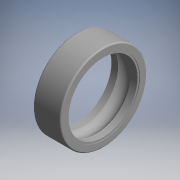
# Autodesk Inventor part: 607ZZ Outer ring
Saved by Autodesk Inventor 2017.3 (Build 213256000, 256)
## iProperties
Part Number: 607ZZ Outer ring
Material: Generic
Catalog Web Link: www.cadenas.de
Description: Six types or-Metric system sizes
Vendor: NTN
Document SubType Name: Modeling
Designer: partserver
Manufacturer: NTN
Mass: 0.543098 g
Surface Area: 8.65362 cm^2
Volume: 0.543098 cm^3
Density: 1 g/cm^3
Appearance: PSOLRGB-192-192-192
Category: PARTsolutions
Company: NTN
Title: 607ZZ Outer ring
Author: Cadenas PARTsolutions
Comments: Metric system sizes
PSOL_IDENT_0: {$CADENAS_DATA\23d-libs\ntn\ball_roller_bearings\miniature_extra_small_bb\metric_system_sizes\mss_or
PSOL_IDENT_1: .prj},181 {VTYP=3D},{NB=607ZZ Outer ring},{LINA=607ZZ Outer ring},{NN=Six types or},{DATE=21.12.2021
PSOL_IDENT_2: 04:23:05},{GEOMDATE=06.03.2020 10:07:12},{VERSION=},{LINEID=12950},{WBVAR=},{WBNUMERIC=}  {NB=607ZZ
PSOL_IDENT_3: Outer ring},{LINA=607ZZ Outer ring},{KT=DUMMY},{IDNR=},{SD=7.0},{D=19},{B=6.0},{R=0.30},{ORDER=607Z
PSOL_IDENT_4: Z},{CR=2 240},{COR=910},{CRF=228},{CORF=93},{LSG=34 000},{LSO=40 000},{MASS=8.00},{D1=0.0},{D2=0.0},
PSOL_IDENT_5: {C1=0.0},{C2=0.0},{ORDER1=607},{WSS=607ZZ},{WDS=ZZ},{UTWF=0},{FORSS=0},{FORDS=0},{DA1=9},{DA2=10,4},
PSOL_IDENT_6: {DA=17},{RAS=0,3},{MASS1=0.00},{B1=6.0},{VERS=3},{X=6},{N=7},{O=40.82},{RB=1.776}
NB: 607ZZ Outer ring
NN: Six types or
NT: Metric system sizes
NBSYN: $ORDER. Outer ring
LINA: 607ZZ Outer ring
CATALOG: NTN Corporation
SD: 7
D: 19
B: 6
R: 0.3
CR: 2 240
COR: 910
CRF: 228
CORF: 93
LSG: 34 000
LSO: 40 000
MASS: 8
D1: 0
D2: 0
C1: 0
C2: 0
ORDER1: 607
WSS: 607ZZ
WDS: ZZ
UTWF: 0
FORSS: 0
FORDS: 0
DA1: 9
DA2: 10,4
DA: 17
RAS: 0,3
MASS1: 0
B1: 6
VERS: 3
SUPPLIER: NTN
ARTICLENO: 607ZZ Outer ring
BOMINFO: 607ZZ Outer ring
CREATOR: CADENAS GmbH
Autodesk Inventor part; units mm, degrees
sketch "Sketch_3" plane through (0, 0, 0) normal (0, 0, 1) x (1, 0, 0)
  line L0 (6, 0) -> (0, 0)
  line L1 (0, 7.964) -> (0.135, 7.964)
  line L2 (0.135, 7.964) -> (0.135, 7.58)
  line L3 (0.135, 7.58) -> (1.5901, 7.58)
  arc A0 (4.4099, 7.58) -> (1.5901, 7.58) centre (3, 6.5) ccw
  line L4 (4.4099, 7.58) -> (5.865, 7.58)
  line L5 (5.865, 7.58) -> (5.865, 7.964)
  line L6 (5.865, 7.964) -> (6, 7.964)
  line L7 (6, 7.964) -> (6, 9.2)
  arc A1 (6, 9.2) -> (5.7, 9.5) centre (5.7, 9.2) ccw
  line L8 (5.7, 9.5) -> (0.3, 9.5)
  arc A2 (0.3, 9.5) -> (0, 9.2) centre (0.3, 9.2) ccw
  line L9 (0, 9.2) -> (0, 7.964)
  constraints: 20 end point, 6 point on circle, 3 centre point
revolve "Revolution1" add sketch "Sketch_3" angle 360 about axis through (6, 0, 0) along (1, 0, 0)
ref_plane "mss_or_XY" through (0, 0, 0) normal (1, 0, 0) x (0, 0, -1)
ref_plane "mss_or_YZ" through (0, 0, 0) normal (0, 0, -1) x (0, 1, 0)
ref_plane "mss_or_ZX" through (0, 0, 0) normal (0, 1, 0) x (1, 0, 0)
ref_plane "mss_or11_XY" through (6, 0, 0) normal (1, 0, 0) x (0, 0, -1)
ref_plane "mss_or11_YZ" through (6, 0, 0) normal (0, 0, -1) x (0, 1, 0)
ref_plane "mss_or11_ZX" through (6, 0, 0) normal (0, 1, 0) x (1, 0, 0)
ref_plane "mss_or2_1_XY" through (3, 6.5, 0) normal (1, 0, 0) x (0, 0, -1)
ref_plane "mss_or2_1_YZ" through (3, 6.5, 0) normal (0, 0, -1) x (0, 1, 0)
ref_plane "mss_or2_1_ZX" through (3, 6.5, 0) normal (0, 1, 0) x (1, 0, 0)
ref_plane "mss_or2_2_XY" through (3, 4.0527, 5.0819) normal (1, 0, 0) x (0, 0, -1)
ref_plane "mss_or2_2_YZ" through (3, 4.0527, 5.0819) normal (0, 0, -1) x (0, 1, 0)
ref_plane "mss_or2_2_ZX" through (3, 4.0527, 5.0819) normal (0, 1, 0) x (1, 0, 0)
ref_plane "mss_or2_3_XY" through (3, -1.4464, 6.337) normal (1, 0, 0) x (0, 0, -1)
ref_plane "mss_or2_3_YZ" through (3, -1.4464, 6.337) normal (0, 0, -1) x (0, 1, 0)
ref_plane "mss_or2_3_ZX" through (3, -1.4464, 6.337) normal (0, 1, 0) x (1, 0, 0)
ref_plane "mss_or2_4_XY" through (3, -5.8563, 2.8202) normal (1, 0, 0) x (0, 0, -1)
ref_plane "mss_or2_4_YZ" through (3, -5.8563, 2.8202) normal (0, 0, -1) x (0, 1, 0)
ref_plane "mss_or2_4_ZX" through (3, -5.8563, 2.8202) normal (0, 1, 0) x (1, 0, 0)
ref_plane "mss_or2_5_XY" through (3, -5.8563, -2.8202) normal (1, 0, 0) x (0, 0, -1)
ref_plane "mss_or2_5_YZ" through (3, -5.8563, -2.8202) normal (0, 0, -1) x (0, 1, 0)
ref_plane "mss_or2_5_ZX" through (3, -5.8563, -2.8202) normal (0, 1, 0) x (1, 0, 0)
ref_plane "mss_or2_6_XY" through (3, -1.4464, -6.337) normal (1, 0, 0) x (0, 0, -1)
ref_plane "mss_or2_6_YZ" through (3, -1.4464, -6.337) normal (0, 0, -1) x (0, 1, 0)
ref_plane "mss_or2_6_ZX" through (3, -1.4464, -6.337) normal (0, 1, 0) x (1, 0, 0)
ref_plane "mss_or2_7_XY" through (3, 4.0527, -5.0819) normal (1, 0, 0) x (0, 0, -1)
ref_plane "mss_or2_7_YZ" through (3, 4.0527, -5.0819) normal (0, 0, -1) x (0, 1, 0)
ref_plane "mss_or2_7_ZX" through (3, 4.0527, -5.0819) normal (0, 1, 0) x (1, 0, 0)
ref_plane "mss_or21_1_XY" through (3, 6.5, 0) normal (1, 0, 0) x (0, 0, -1)
ref_plane "mss_or21_1_YZ" through (3, 6.5, 0) normal (0, 0, -1) x (0, 1, 0)
ref_plane "mss_or21_1_ZX" through (3, 6.5, 0) normal (0, 1, 0) x (1, 0, 0)
ref_plane "mss_or21_2_XY" through (3, 4.0527, 5.0819) normal (1, 0, 0) x (0, 0, -1)
ref_plane "mss_or21_2_YZ" through (3, 4.0527, 5.0819) normal (0, 0, -1) x (0, 1, 0)
ref_plane "mss_or21_2_ZX" through (3, 4.0527, 5.0819) normal (0, 1, 0) x (1, 0, 0)
ref_plane "mss_or21_3_XY" through (3, -1.4464, 6.337) normal (1, 0, 0) x (0, 0, -1)
ref_plane "mss_or21_3_YZ" through (3, -1.4464, 6.337) normal (0, 0, -1) x (0, 1, 0)
ref_plane "mss_or21_3_ZX" through (3, -1.4464, 6.337) normal (0, 1, 0) x (1, 0, 0)
ref_plane "mss_or21_4_XY" through (3, -5.8563, 2.8202) normal (1, 0, 0) x (0, 0, -1)
ref_plane "mss_or21_4_YZ" through (3, -5.8563, 2.8202) normal (0, 0, -1) x (0, 1, 0)
ref_plane "mss_or21_4_ZX" through (3, -5.8563, 2.8202) normal (0, 1, 0) x (1, 0, 0)
ref_plane "mss_or21_5_XY" through (3, -5.8563, -2.8202) normal (1, 0, 0) x (0, 0, -1)
ref_plane "mss_or21_5_YZ" through (3, -5.8563, -2.8202) normal (0, 0, -1) x (0, 1, 0)
ref_plane "mss_or21_5_ZX" through (3, -5.8563, -2.8202) normal (0, 1, 0) x (1, 0, 0)
ref_plane "mss_or21_6_XY" through (3, -1.4464, -6.337) normal (1, 0, 0) x (0, 0, -1)
ref_plane "mss_or21_6_YZ" through (3, -1.4464, -6.337) normal (0, 0, -1) x (0, 1, 0)
ref_plane "mss_or21_6_ZX" through (3, -1.4464, -6.337) normal (0, 1, 0) x (1, 0, 0)
ref_plane "mss_or21_7_XY" through (3, 4.0527, -5.0819) normal (1, 0, 0) x (0, 0, -1)
ref_plane "mss_or21_7_YZ" through (3, 4.0527, -5.0819) normal (0, 0, -1) x (0, 1, 0)
ref_plane "mss_or21_7_ZX" through (3, 4.0527, -5.0819) normal (0, 1, 0) x (1, 0, 0)
body "Solid1"
